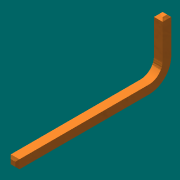
# Autodesk Inventor part: PinRight2
Saved by Autodesk Inventor 2016 SP1 (Build 200210100, 210)
## iProperties
Created: 2014-07-19
Part Number: PinRight2
Material: Gold
Document SubType Name: Modeling
Designer: Sawaiz Syed
Density: 19.3 g/cm^3
Appearance: Metal 1600F Hot
Author: Sawaiz Syed
Autodesk Inventor part; units mm, degrees
note: some values were not read from the file. Chosen so that the rebuilt part matches the saved one: bend side of "Bend Part1".
ref_plane "YZ Plane" through (0, 0, 0) normal (1, 0, 0) x (0, 1, 0)
ref_plane "XZ Plane" through (0, 0, 0) normal (0, 1, 0) x (-1, 0, 0)
ref_plane "XY Plane" through (0, 0, 0) normal (0, 0, 1) x (1, 0, 0)
sketch "Sketch1" plane through (0, 0, 0) normal (0, 1, 0) x (-1, 0, 0)
  line L0 (0.32, -0.32) -> (-0.32, -0.32)
  line L1 (-0.32, -0.32) -> (-0.32, 0.32)
  line L2 (-0.32, 0.32) -> (0.32, 0.32)
  line L3 (0.32, 0.32) -> (0.32, -0.32)
  line L4 (0.32, -0.32) -> (-0.32, 0.32) construction
  line L5 (-0.32, -0.32) -> (0.32, 0.32) construction
  point P0 (0, 0)
  dimension "d0" = 0.64
  dimension "d1" = 0.64
  constraints: 12 end point, 2 midpoint, 2 parallel, 1 horizontal, 1 perpendicular
  measures "d0" distance of L1.end L2.end
  measures "d1" distance of L0.end L1.end
extrude "Extrusion1" add sketch "Sketch1" along normal blind 14.0176
chamfer "Chamfer1" distance 0.155 angle 45 8 edges at (0.32, 14.0176, 0) (0, 14.0176, -0.32) (0, 14.0176, 0.32) (-0.32, 14.0176, 0) (0.32, 0, 0) (0, 0, -0.32) (0, 0, 0.32) (-0.32, 0, 0)
sketch "Sketch2" plane through (-0.32, 0.155, 0.32) normal (0, 0, 1) x (1, 0, 0)
  line L0 (-0.9237, 9.6188) -> (1.8536, 9.6188)
  point P0 (0.32, -0.155)
  dimension "d7" = 9.7738
  constraints: 2 end point, 1 horizontal
  measures "d7" distance from line of point (0.32, -0.155) L0
bend part "Bend Part1" radius 1 angle 90 line through (-1.2437, 9.7738, 0.32) along (1, 0, 0) centre toward (0, 0, 1) moving side (0, 1, 0) both sides no
body "Solid1"
